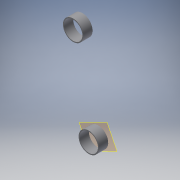
# Autodesk Inventor part: washer connector
Saved by Autodesk Inventor 2019 (Build 230136000, 136)
## iProperties
Created: 2018-10-09
Part Number: washer connector
Material: Generic
Document SubType Name: Modeling
Designer: HIVE
Density: 1 g/cm^3
Appearance: Default
Author: HIVE
Autodesk Inventor part; units mm, degrees
ref_plane "YZ Plane" through (0, 0, 0) normal (1, 0, 0) x (0, 1, 0)
ref_plane "XZ Plane" through (0, 0, 0) normal (0, 1, 0) x (-1, 0, 0)
ref_plane "XY Plane" through (0, 0, 0) normal (0, 0, 1) x (1, 0, 0)
sketch "Sketch1" plane through (0, 0, 0) normal (0, 0, 1) x (1, 0, 0)
  circle A0 centre (3.556, 0) radius 8.7376 projected
  circle A1 centre (3.556, 0) radius 7.9439 projected
  point P0 (0, 0)
extrude "Extrusion1" add sketch "Sketch1" along normal blind 4
ref_plane "Work Plane1" through (15.4309, -73.6057, 0) normal (0, 0, 1) x (0.4429, -0.8966, 0)
sketch "Sketch2" plane through (15.4309, -73.6057, 0) normal (0, 0, 1) x (0.4429, -0.8966, 0)
  circle A0 centre (3.556, 0) radius 8.7376 projected
  circle A1 centre (3.556, 0) radius 7.9438 projected
  point P0 (-72.8269, 18.7655)
extrude "Extrusion2" add sketch "Sketch2" along normal blind 4
body "Solid1"
